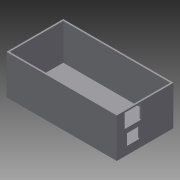
# Autodesk Inventor part: SD_BaseStation_Box
Saved by Autodesk Inventor 2015 (Build 190159000, 159)
## iProperties
Created: 2014-04-30
Part Number: SD_BaseStation_Box
Material: Generic
Document SubType Name: Modeling
Designer: xbmc
Density: 1 g/cm^3
Appearance: Default
Author: xbmc
Autodesk Inventor part; units mm, degrees
ref_plane "YZ Plane" through (0, 0, 0) normal (1, 0, 0) x (0, 1, 0)
ref_plane "XZ Plane" through (0, 0, 0) normal (0, 1, 0) x (-1, 0, 0)
ref_plane "XY Plane" through (0, 0, 0) normal (0, 0, 1) x (1, 0, 0)
sketch "Sketch1" plane through (0, 0, 0) normal (0, 1, 0) x (-1, 0, 0)
  line L0 (1.6318, 52.1856) -> (-109.4932, 52.1856)
  line L1 (-109.4932, 52.1856) -> (-109.4932, -4.9644)
  line L2 (-109.4932, -4.9644) -> (1.6318, -4.9644)
  line L3 (1.6318, -4.9644) -> (1.6318, 52.1856)
  point P0 (0, 0)
  constraints: 8 end point, 2 parallel, 1 horizontal, 1 perpendicular
extrude "Extrusion1" add sketch "Sketch1" along normal blind 39.6875
sketch "Sketch2" plane through (0, 39.6875, 0) normal (0, 1, 0) x (1, 0, 0)
  line L0 (-0.0443, -50.5981) -> (107.9057, -50.5981)
  line L1 (107.9057, -50.5981) -> (107.9057, 3.3769)
  line L2 (107.9057, 3.3769) -> (-0.0443, 3.3769)
  line L3 (-0.0443, 3.3769) -> (-0.0443, -50.5981)
  line L4 (-1.6318, -52.1856) -> (109.4932, -52.1856) projected
  line L5 (109.4932, 4.9644) -> (-1.6318, 4.9644) projected
  line L6 (-1.6318, 4.9644) -> (-1.6318, -52.1856) projected
  line L7 (109.4932, -52.1856) -> (109.4932, 4.9644) projected
  point P0 (0, 0)
  dimension "d8" = 1.5875
  dimension "d9" = 1.5875
  dimension "d10" = 1.5875
  dimension "d11" = 1.5875
  constraints: 8 end point, 2 parallel, 1 horizontal, 1 perpendicular
  measures "d8" distance between parallel lines of L4 L0
  measures "d9" distance between parallel lines of L5 L2
  measures "d10" distance between parallel lines of L6 L3
  measures "d11" distance between parallel lines of L7 L1
extrude "Extrusion2" cut sketch "Sketch2" against normal blind 36.5125 contours L3 L2 L1 L0
sketch "Sketch3" plane through (109.4932, 0, 52.1856) normal (1, 0, 0) x (0, 0, -1)
  line L0 (10.3187, 19.05) -> (23.0187, 19.05)
  line L1 (23.0187, 19.05) -> (23.0187, 7.9375)
  line L2 (23.0187, 7.9375) -> (10.3187, 7.9375)
  line L3 (10.3187, 7.9375) -> (10.3187, 19.05)
  line L4 (0, 0) -> (57.15, 0) projected
  line L5 (0, 0) -> (0, 39.6875) projected
  line L6 (7.9375, 38.1) -> (24.6062, 38.1)
  line L7 (24.6062, 38.1) -> (24.6062, 23.8125)
  line L8 (24.6062, 23.8125) -> (7.9375, 23.8125)
  line L9 (7.9375, 23.8125) -> (7.9375, 38.1)
  line L10 (0, 39.6875) -> (57.15, 39.6875) projected
  line L11 (55.5625, 3.175) -> (1.5875, 3.175) projected
  line L12 (1.5875, 39.6875) -> (1.5875, 3.175) projected
  point P0 (52.1856, 0)
  point P1 (55.5625, 39.6875)
  point P2 (1.5875, 0)
  dimension "d14" = 12.7
  dimension "d15" = 11.1125
  dimension "d18" = 16.6687
  dimension "d19" = 14.2875
  dimension "d23" = 4.7625
  dimension "d28" = 4.7625
  dimension "d29" = 8.7312
  dimension "d30" = 6.35
  dimension "d34" = 1.5875
  constraints: 16 end point, 4 parallel, 2 horizontal, 2 perpendicular
  measures "d14" distance of L1.end L2.end
  measures "d15" distance of L0.end L1.end
  measures "d18" distance of L7.end L8.end
  measures "d19" distance of L6.end L7.end
  measures "d23" distance between parallel lines of L0 L8
  measures "d28" distance between parallel lines of L11 L2
  measures "d29" distance between parallel lines of L12 L3
  measures "d30" distance between parallel lines of L12 L9
  measures "d34" distance between parallel lines of L10 L6
extrude "Extrusion3" cut sketch "Sketch3" against normal up to surface (1.5875 mm away)
body "Solid1"
